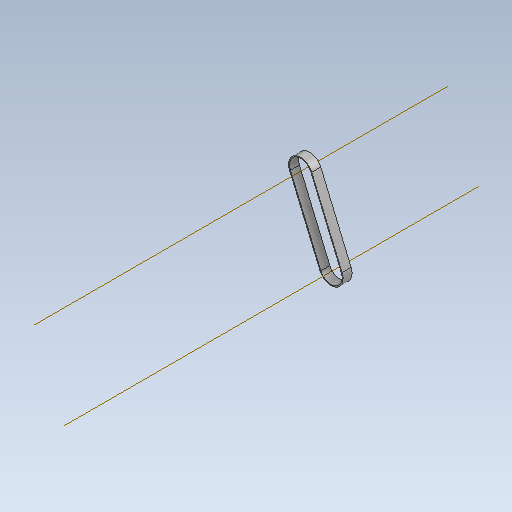
# Autodesk Inventor part: Synchronous Belt
Saved by Autodesk Inventor 2020.3 (Build 243373000, 373)
## iProperties
CustomPartVersion: 1
Created: 2022-07-18
Part Number: Synchronous Belt
Material: Rubber
Document SubType Name: Modeling
Designer: karimi2
Density: 0.93 g/cm^3
Appearance: Rubber - Black - Version 1.1
Mass: 0.603966 g
Surface Area: 22.4998 cm^2
Volume: 0.649426 cm^3
Author: karimi2
Autodesk Inventor part; units mm, degrees
sketch "Sketch Path" plane through (0, 0, 0) normal (0, 0, 1) x (1, 0, 0)
  arc A0 (37.9018, -65.6735) -> (23.0108, -71.9768) centre (30.4563, -68.8251) ccw
  arc A1 (44.423, -122.5611) -> (59.314, -116.2578) centre (51.8685, -119.4094) ccw
  line L0 (44.423, -122.5611) -> (23.0108, -71.9768)
  line L1 (37.9018, -65.6735) -> (59.314, -116.2578)
  constraints: 4 end point, 4 point on circle, 2 centre point
ref_plane "Cross Section Plane" through (23.0108, -71.9768, 0) normal (0.3898, -0.9209, 0) x (0, 0, 1)
ref_plane "Work Plane2" through (30.4563, -68.8251, 0) normal (-1, 0, 0) x (0, 0, 1)
ref_plane "Work Plane3" through (51.8685, -119.4094, 0) normal (-0.3167, 0.9485, 0) x (0, 0, 1)
sketch "Cross Section" plane through (23.0108, -71.9768, 0) normal (0.3898, -0.9209, 0) x (0, 0, 1)
  line L0 (-3.175, 0.381) -> (3.175, 0.381)
  line L1 (3.175, 0.381) -> (3.175, -0.254)
  line L2 (3.175, -0.254) -> (-3.175, -0.254)
  line L3 (-3.175, -0.254) -> (-3.175, 0.381)
  line L4 (-3.175, 0) -> (3.175, 0) construction
  point P0 (0, 0)
  point P1 (0, 0)
  dimension "d0" = 6.35
  dimension "d4" = 0.254
  dimension "d5" = 0.381
  constraints: 10 end point, 2 parallel, 2 point on line, 1 coincident, 1 horizontal, 1 midpoint, 1 perpendicular, 1 other
  measures "d0" distance between parallel lines of L1 L3
  measures "d4" distance between parallel lines of L2 L4
  measures "d5" distance between parallel lines of L4 L0
sweep "Belt" add profiles "Cross Section" path "Sketch Path"
equation "\"d0\" = da_B"
equation "\"d4\" = da_a"
equation "\"d5\" = da_a2"
equation "\"da_B\" = 6.35"
equation "\"da_pb\" = 2.032"
equation "\"da_L\" = 160.659"
equation "\"da_a\" = 0.254"
equation "\"da_S\" = 1.143"
equation "\"da_Beta\" = 20deg"
equation "\"da_Ht\" = 0.508"
equation "\"da_H\" = 1.143"
equation "\"da_a2\" = 0.381"
body "Solid1"
